Internal Limit Switch Holder - Right_v4 (Autodesk Fusion 360 design; units mm, degrees)
Autodesk Fusion 360 part; units mm, degrees
note: some values were not read from the file. Set by a fixed rule: which sketch regions a step uses.
sketch "Sketch1" plane through (0, 0, 0) normal (0, 0, 1) x (1, 0, 0)
  line L0 (10, 4.8314) -> (10, 9.5)
  line L1 (-4.4022, -9.8222) -> (-3.1214, -8.5414)
  arc A0 (3.2628, -8.2) -> (3.1214, -8.5414) centre (3.2628, -8.4) ccw
  line L2 (-5.5, 6.5607) -> (-5.5, 8.2)
  line L3 (-5.5, -6.5607) -> (-2.8393, -3.9)
  line L4 (-4.8314, 10) -> (-9.5, 10)
  line L5 (2.8393, 3.9) -> (-2.8393, 3.9)
  arc A1 (-10, -9.5) -> (-9.5, -10) centre (-9.5, -9.5) ccw
  line L6 (9.5, 10) -> (4.8314, 10)
  arc A2 (-3.2628, 8.2) -> (-3.1214, 8.5414) centre (-3.2628, 8.4) ccw
  line L7 (-8.2, 3.2628) -> (-8.2, 5.5)
  line L8 (2.8393, -3.9) -> (5.5, -6.5607)
  line L9 (-10, 9.5) -> (-10, 4.9)
  arc A3 (9.5, -10) -> (10, -9.5) centre (9.5, -9.5) ccw
  line L10 (-6.5607, -5.5) -> (-8.2, -5.5)
  line L11 (3.1214, -8.5414) -> (4.2336, -9.6536)
  line L12 (-8.2, -5.5) -> (-8.2, -3.2628)
  line L13 (-9.9987, -4.7917) -> (-10, -9.5)
  line L14 (10, -9.5) -> (10, -4.8314)
  line L15 (3.2628, 8.2) -> (5.5, 8.2)
  arc A4 (8.5414, -3.1214) -> (8.2, -3.2628) centre (8.4, -3.2628) ccw
  arc A5 (-3.1214, -8.5414) -> (-3.2628, -8.2) centre (-3.2628, -8.4) ccw
  line L16 (4.8314, -10) -> (9.5, -10)
  line L17 (-3.9, -2.8393) -> (-6.5607, -5.5)
  line L18 (-3.2628, -8.2) -> (-5.5, -8.2)
  line L19 (3.9, 2.8393) -> (6.5607, 5.5)
  line L20 (-3.1214, 8.5414) -> (-4.4312, 9.8494)
  line L21 (8.2, -5.5) -> (6.5607, -5.5)
  arc A6 (-10, 4.9) -> (-9.8494, 4.4312) centre (-9.3734, 4.8428) ccw
  line L22 (8.5414, 3.1214) -> (9.8222, 4.4022)
  circle A7 centre (0, 0) radius 2.1
  line L23 (3.9, -2.8393) -> (3.9, 2.8393)
  line L24 (6.5607, -5.5) -> (3.9, -2.8393)
  line L25 (5.5, -6.5607) -> (5.5, -8.2)
  line L26 (8.2, -3.2628) -> (8.2, -5.5)
  arc A8 (10, -4.8314) -> (9.8222, -4.4022) centre (9.3929, -4.8314) ccw
  line L27 (-5.5, -8.2) -> (-5.5, -6.5607)
  arc A9 (-4.8314, -10) -> (-4.4022, -9.8222) centre (-4.8314, -9.3929) ccw
  line L28 (5.5, -8.2) -> (3.2628, -8.2)
  line L29 (9.8222, -4.4022) -> (8.5414, -3.1214)
  arc A10 (-9.8222, -4.4022) -> (-9.9987, -4.7917) centre (-9.3929, -4.8314) ccw
  line L30 (-8.5414, -3.1214) -> (-9.8222, -4.4022)
  arc A11 (4.2336, -9.6536) -> (4.8314, -10) centre (4.8837, -9.2207) ccw
  arc A12 (-8.2, -3.2628) -> (-8.5414, -3.1214) centre (-8.4, -3.2628) ccw
  line L31 (-9.5, -10) -> (-4.8314, -10)
  line L32 (-2.8393, -3.9) -> (2.8393, -3.9)
  line L33 (-5.8557, 10) -> (6.4454, 10) construction
  arc A13 (10, 9.5) -> (9.5, 10) centre (9.5, 9.5) ccw
  arc A14 (3.1214, 8.5414) -> (3.2628, 8.2) centre (3.2628, 8.4) ccw
  line L34 (-5.5, 8.2) -> (-3.2628, 8.2)
  line L35 (-3.9, 2.8393) -> (-3.9, -2.8393)
  line L36 (4.4022, 9.8222) -> (3.1214, 8.5414)
  arc A15 (4.8314, 10) -> (4.4022, 9.8222) centre (4.8314, 9.3929) ccw
  line L37 (-9.8494, 4.4312) -> (-8.5414, 3.1214)
  line L38 (5.5, 8.2) -> (5.5, 6.5607)
  line L39 (6.5607, 5.5) -> (8.2, 5.5)
  arc A16 (-8.5414, 3.1214) -> (-8.2, 3.2628) centre (-8.4, 3.2628) ccw
  line L40 (8.2, 5.5) -> (8.2, 3.2628)
  arc A17 (-4.4312, 9.8494) -> (-4.8314, 10) centre (-4.8314, 9.3929) ccw
  line L41 (-8.2, 5.5) -> (-6.5607, 5.5)
  arc A18 (9.8222, 4.4022) -> (10, 4.8314) centre (9.3929, 4.8314) ccw
  arc A19 (-9.5, 10) -> (-10, 9.5) centre (-9.5, 9.5) ccw
  line L42 (-2.8393, 3.9) -> (-5.5, 6.5607)
  line L43 (-6.5607, 5.5) -> (-3.9, 2.8393)
  arc A20 (8.2, 3.2628) -> (8.5414, 3.1214) centre (8.4, 3.2628) ccw
  line L44 (5.5, 6.5607) -> (2.8393, 3.9)
  line L45 (5.4, -6.6021) -> (5.4, -8.1)
  line L46 (5.4, -8.1) -> (3.2628, -8.1)
  arc A21 (3.2628, -8.1) -> (3.0507, -8.6121) centre (3.2628, -8.4) ccw
  line L47 (3.0507, -8.6121) -> (4.1561, -9.7175)
  arc A22 (4.1561, -9.7175) -> (4.8282, -10.1) centre (4.8837, -9.2207) ccw
  line L48 (4.8282, -10.1) -> (9.5, -10.1)
  arc A23 (9.5, -10.1) -> (10.1, -9.5) centre (9.5, -9.5) ccw
  line L49 (10.1, -9.5) -> (10.1, -4.8314)
  arc A24 (10.1, -4.8314) -> (9.8929, -4.3315) centre (9.3929, -4.8314) ccw
  line L50 (9.8929, -4.3315) -> (8.6121, -3.0507)
  arc A25 (8.6121, -3.0507) -> (8.1, -3.2628) centre (8.4, -3.2628) ccw
  line L51 (8.1, -3.2628) -> (8.1, -5.4)
  line L52 (8.1, -5.4) -> (6.6021, -5.4)
  line L53 (6.6021, -5.4) -> (4, -2.7979)
  line L54 (4, -2.7979) -> (4, 2.7979)
  line L55 (4, 2.7979) -> (6.6021, 5.4)
  line L56 (6.6021, 5.4) -> (8.1, 5.4)
  line L57 (8.1, 5.4) -> (8.1, 3.2628)
  arc A26 (8.1, 3.2628) -> (8.6121, 3.0507) centre (8.4, 3.2628) ccw
  line L58 (8.6121, 3.0507) -> (9.8929, 4.3315)
  arc A27 (9.8929, 4.3315) -> (10.1, 4.8314) centre (9.3929, 4.8314) ccw
  line L59 (10.1, 4.8314) -> (10.1, 9.5)
  arc A28 (10.1, 9.5) -> (9.5, 10.1) centre (9.5, 9.5) ccw
  line L60 (9.5, 10.1) -> (4.8314, 10.1)
  arc A29 (4.8314, 10.1) -> (4.3315, 9.8929) centre (4.8314, 9.3929) ccw
  line L61 (4.3315, 9.8929) -> (3.0507, 8.6121)
  arc A30 (3.0507, 8.6121) -> (3.2628, 8.1) centre (3.2628, 8.4) ccw
  line L62 (3.2628, 8.1) -> (5.4, 8.1)
  line L63 (5.4, 8.1) -> (5.4, 6.6021)
  line L64 (5.4, 6.6021) -> (2.7979, 4)
  line L65 (2.7979, 4) -> (-2.7979, 4)
  line L66 (-2.7979, 4) -> (-5.4, 6.6021)
  line L67 (-5.4, 6.6021) -> (-5.4, 8.1)
  line L68 (-5.4, 8.1) -> (-3.2628, 8.1)
  arc A31 (-3.2628, 8.1) -> (-3.0509, 8.6124) centre (-3.2628, 8.4) ccw
  line L69 (-3.0509, 8.6124) -> (-4.3627, 9.9223)
  arc A32 (-4.3627, 9.9223) -> (-4.8314, 10.1) centre (-4.8314, 9.3929) ccw
  line L70 (-4.8314, 10.1) -> (-9.5, 10.1)
  arc A33 (-9.5, 10.1) -> (-10.1, 9.5) centre (-9.5, 9.5) ccw
  line L71 (-10.1, 9.5) -> (-10.1, 4.9044)
  arc A34 (-10.1, 4.9044) -> (-9.9226, 4.363) centre (-9.3734, 4.8428) ccw
  line L72 (-9.9226, 4.363) -> (-8.6124, 3.0509)
  arc A35 (-8.6124, 3.0509) -> (-8.1, 3.2628) centre (-8.4, 3.2628) ccw
  line L73 (-8.1, 3.2628) -> (-8.1, 5.4)
  line L74 (-8.1, 5.4) -> (-6.6021, 5.4)
  line L75 (-6.6021, 5.4) -> (-4, 2.7979)
  line L76 (-4, 2.7979) -> (-4, -2.7979)
  line L77 (-4, -2.7979) -> (-6.6021, -5.4)
  line L78 (-6.6021, -5.4) -> (-8.1, -5.4)
  line L79 (-8.1, -5.4) -> (-8.1, -3.2628)
  arc A36 (-8.1, -3.2628) -> (-8.6121, -3.0507) centre (-8.4, -3.2628) ccw
  line L80 (-8.6121, -3.0507) -> (-9.8929, -4.3315)
  arc A37 (-9.8929, -4.3315) -> (-10.0987, -4.7886) centre (-9.3929, -4.8314) ccw
  line L81 (-10.0987, -4.7886) -> (-10.1, -9.4997)
  arc A38 (-10.1, -9.4997) -> (-9.5, -10.1) centre (-9.5, -9.5) ccw
  line L82 (-9.5, -10.1) -> (-4.8314, -10.1)
  arc A39 (-4.8314, -10.1) -> (-4.3315, -9.8929) centre (-4.8314, -9.3929) ccw
  line L83 (-4.3315, -9.8929) -> (-3.0507, -8.6121)
  arc A40 (-3.0507, -8.6121) -> (-3.2628, -8.1) centre (-3.2628, -8.4) ccw
  line L84 (-3.2628, -8.1) -> (-5.4, -8.1)
  line L85 (-5.4, -8.1) -> (-5.4, -6.6021)
  line L86 (-5.4, -6.6021) -> (-2.7979, -4)
  line L87 (-2.7979, -4) -> (2.7979, -4)
  line L88 (2.7979, -4) -> (5.4, -6.6021)
  line L89 (-9.5, -9.5) -> (9.5, -9.5)
  line L90 (9.5, -9.5) -> (9.5, -17.5)
  line L91 (9.5, -17.5) -> (-9.5, -17.5)
  line L92 (-9.5, -17.5) -> (-9.5, -9.5)
  dimension "d1" = 0.1
  dimension "d2" = 8
  constraint coincident L33.start L4
  constraint coincident L33.end L6
  constraint horizontal L89
  constraint vertical L90
  constraint horizontal L91
  constraint vertical L92
  constraint coincident A1.centre A38.centre
  measures "d2" distance of A1.centre L91.end
extrude "Extrude1" add sketch "Sketch1" along normal blind 35 contours L47 A22 L48 L82 A39 L83 L89 L90 L91 L92 | L45 L46 A21 L47 L83 A40 L84 L85 L86 L87 L88 L89
sketch "Sketch2" plane through (0, -17.5, 0) normal (0, -1, 0) x (1, 0, 0)
  line L0 (-9.5, 0) -> (9.5, 0)
  line L1 (9.5, 0) -> (9.5, 35)
  line L2 (9.5, 35) -> (-9.5, 35)
  line L3 (-9.5, 35) -> (-9.5, 0)
  line L4 (13.7568, 12.4504) -> (-13.7568, 12.5496) construction
  line L5 (0.3182, 26.2532) -> (13.7532, 12.8182)
  line L6 (13.7532, 12.8182) -> (-0.3182, -1.2532)
  line L7 (-0.3182, -1.2532) -> (-13.7532, 12.1818)
  line L8 (-13.7532, 12.1818) -> (0.3182, 26.2532)
  line L9 (0.3182, 26.2532) -> (-0.3182, -1.2532) construction
  line L10 (13.7532, 12.8182) -> (-13.7532, 12.1818) construction
  line L11 (-13.7532, 12.1818) -> (-8.3085, 6.7371) construction
  line L12 (-8.3085, 6.7371) -> (5.7629, 20.8085) construction
  line L13 (-8.3085, 6.7371) -> (-4.6669, 10.3787) construction
  line L14 (-4.6669, 10.3787) -> (2.1213, 17.1669) construction
  line L15 (2.1213, 17.1669) -> (5.7629, 20.8085) construction
  line L16 (2.1213, 17.1669) -> (5.7629, 20.8085) construction
  circle A0 centre (2.1213, 17.1669) radius 1.05
  circle A1 centre (-4.6669, 10.3787) radius 1.05
  line L17 (0.3182, 26.2532) -> (-8.4286, 35)
  point P0 (0, 12.5)
  dimension "d15" = 19.9
  dimension "d16" = 7.7
  dimension "d17" = 5.15
  dimension "d18" = 9.6
  dimension "d19" = 5.15
  dimension "d20" = 2.1
  dimension "d21" = 2.1
  constraint perpendicular L5 L6
  constraint parallel L5 L7
  constraint parallel L6 L8
  constraint coincident L9 P0
  constraint coincident L10 P0
  constraint perpendicular L8 L11
  constraint coincident L5 L12.end
  constraint perpendicular L5 L12
  constraint coincident L12 L13.end
  constraint parallel L12 L14
  constraint perpendicular L5 L16
  constraint coincident L14.end L15.start
  constraint coincident L13.end L14.start
  constraint coincident L2 L17.end
  constraint perpendicular L8 L17
  measures "d15" distance of L5.end L6.end
  measures "d16" distance of L7.end L11.end
  measures "d17" distance of L11.end L13.end
  measures "d18" distance of L13.end L14.end
  measures "d19" distance of L14.end L12.end
  measures "d20" diameter of A0
  measures "d21" diameter of A1
extrude "Extrude2" cut sketch "Sketch2" against normal blind 6.5 contours L0 L1 L3 L5 L6 L7 L8 | L0 L1 L6 | L2 L3 L8 L17
sketch "Sketch3" plane through (0, -17.5, 0) normal (0, -1, 0) x (1, 0, 0)
  line L0 (-8.4286, 35) -> (9.5, 17.0714)
  line L1 (9.5, 17.0714) -> (9.5, 35)
  line L2 (9.5, 35) -> (-8.4286, 35)
  line L3 (9.5, 35) -> (0, 35) construction
  circle A0 centre (0, 31.6) radius 1.55
  circle A1 centre (0, 31.6) radius 3
  dimension "d22" = 3.1
  dimension "d23" = 6
  constraint coincident L1.end L2.start
  constraint coincident L2 L3.end
  constraint concentric A0 A1
  measures "d22" diameter of A0
  measures "d23" diameter of A1
extrude "Extrude3" cut sketch "Sketch3" against normal blind 20 contours A0
extrude "Extrude4" cut sketch "Sketch3" against normal blind 3 contours A1
sketch "Sketch4" plane through (0, 0, 35) normal (0, 0, 1) x (-1, 0, 0)
  line L0 (8.4286, 11) -> (8.4286, 17.5)
  line L1 (8.4286, 17.5) -> (-9.5, 17.5)
  line L2 (-9.5, 17.5) -> (-9.5, 10.1)
  line L3 (-9.5, 10.1) -> (-4.8282, 10.1)
  arc A0 (-4.1561, 9.7175) -> (-4.8282, 10.1) centre (-4.8837, 9.2207) ccw
  line L4 (-4.1561, 9.7175) -> (-3.0507, 8.6121)
  arc A1 (-3.2628, 8.1) -> (-3.0507, 8.6121) centre (-3.2628, 8.4) ccw
  line L5 (-3.2628, 8.1) -> (-5.4, 8.1)
  line L6 (-5.4, 8.1) -> (-5.4, 6.6021)
  line L7 (-5.4, 6.6021) -> (-2.7979, 4)
  line L8 (-2.7979, 4) -> (2.7979, 4)
  line L9 (2.7979, 4) -> (5.4, 6.6021)
  line L10 (5.4, 6.6021) -> (5.4, 8.1)
  line L11 (5.4, 8.1) -> (3.2628, 8.1)
  arc A2 (3.0507, 8.6121) -> (3.2628, 8.1) centre (3.2628, 8.4) ccw
  line L12 (3.0507, 8.6121) -> (4.3315, 9.8929)
  arc A3 (4.8314, 10.1) -> (4.3315, 9.8929) centre (4.8314, 9.3929) ccw
  line L13 (4.8314, 10.1) -> (9.5, 10.1)
  line L14 (9.5, 10.1) -> (9.5, 11)
  line L15 (9.5, 11) -> (8.4286, 11)
  line L16 (0, 4) -> (0, 17.5) construction
  line L17 (2.8, 12.95) -> (-2.8, 12.95)
  line L18 (-2.8, 12.95) -> (-2.8, 11.05)
  line L19 (-2.8, 11.05) -> (2.8, 11.05)
  line L20 (2.8, 11.05) -> (2.8, 12.95)
  line L21 (2.8, 12.95) -> (-2.8, 11.05) construction
  line L22 (-2.8, 12.95) -> (2.8, 11.05) construction
  point P0 (0, 12)
  point P1 (0, 17.5)
  dimension "d28" = 5.6
  dimension "d29" = 1.9
  dimension "d30" = 5.5
  constraint midpoint L8 L16.start
  constraint coincident L1 P1
  constraint perpendicular L1 L16
  constraint horizontal L17
  constraint perpendicular L17 L18
  constraint parallel L17 L19
  constraint parallel L18 L20
  constraint coincident L21 P0
  constraint coincident L22 P0
  constraint coincident L16 P0
  measures "d28" distance of L18.end L19.end
  measures "d29" distance of L17.end L18.end
  measures "d30" distance of P0 P1
extrude "Extrude5" cut sketch "Sketch4" against normal blind 6.5 contours L17 L18 L19 L20
